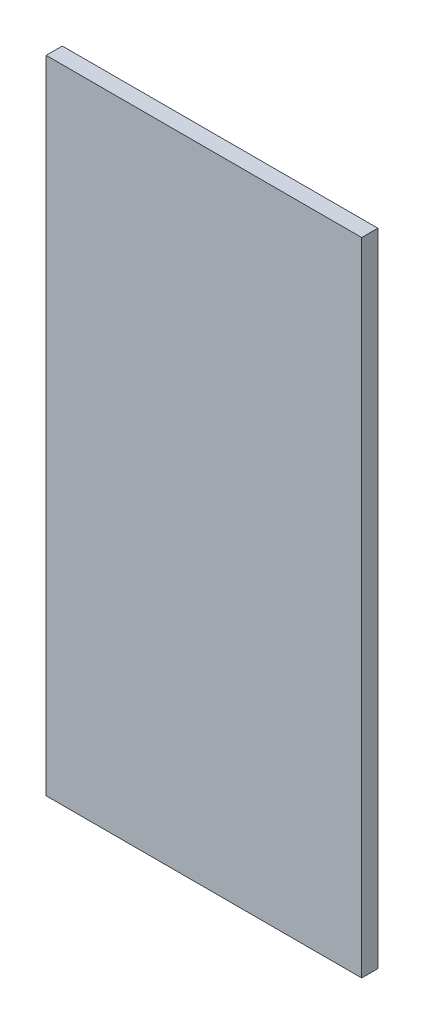
# Autodesk Inventor part: door
Saved by Autodesk Inventor 2023 (Build 270158000, 158)
## iProperties
Created: 2023-04-03
Part Number: door
Material: Generic
Document SubType Name: Modeling
Designer: shrey
Density: 1 g/cm^3
Appearance: Default
Author: shrey
Autodesk Inventor part; units mm, degrees
ref_plane "YZ Plane" through (0, 0, 0) normal (1, 0, 0) x (0, 1, 0)
ref_plane "XZ Plane" through (0, 0, 0) normal (0, 1, 0) x (-1, 0, 0)
ref_plane "XY Plane" through (0, 0, 0) normal (0, 0, 1) x (1, 0, 0)
ref_plane "Work Plane1" through (35.594, 304.8, 19.7663) normal (0, 1, 0) x (-1, 0, 0)
sketch "Sketch1" plane through (35.594, 304.8, 19.7663) normal (0, 1, 0) x (-1, 0, 0)
  line L0 (38.594, -19.7663) -> (338.594, -19.7663)
  line L1 (338.594, -19.7663) -> (338.594, -4.4065)
  line L2 (338.594, -4.4065) -> (38.594, -4.4065)
  line L3 (38.594, -4.4065) -> (38.594, -19.7663)
  line L4 (-28.594, 8.7337) -> (-18.6905, 8.7337) projected
  line L5 (-18.6905, 8.7337) -> (-18.6905, 7.8485) projected
  spline S0 degree 4 poles (-18.6905, 7.8485) (-15.5521, 7.5495) (-7.3401, 9.7663) (-0.7334, 3.3877) (4.6646, 4.702) (6.2676, 4.9792) knots 0 0 0 0 0 0.558486 0.866888 0.866888 0.866888 0.866888 0.866888 projected
  line L6 (6.2676, 4.9792) -> (8.6213, 4.8047) projected
  line L7 (8.6213, 4.8047) -> (8.6213, 3.7665) projected
  line L8 (8.6213, 3.7665) -> (12.5268, 3.3702) projected
  spline S1 degree 2 poles (12.5268, 3.3702) (17.0414, 4.6064) (21.5535, 3.0659) knots 0 0 0 1 1 1 projected
  spline S2 degree 2 poles (21.5535, 3.0659) (24.6084, 3.7058) (28.594, 2.5935) knots 0 0 0 1 1 1 projected
  line L9 (28.594, 2.5935) -> (28.594, -4.4065) projected
  line L10 (28.594, -4.4065) -> (35.594, -4.4065) projected
  line L11 (35.594, -4.4065) -> (35.594, -19.7663) projected
  line L12 (35.594, -19.7663) -> (-139.594, -19.7663) projected
  line L13 (-139.594, -19.7663) -> (-139.594, -9.7663) projected
  line L14 (-139.594, -9.7663) -> (-28.594, -9.7663) projected
  line L15 (-28.594, -9.7663) -> (-28.594, 8.7337) projected
  point P0 (338.594, -12.0864)
  point P1 (38.594, -12.0864)
  dimension "d0" = 3
  dimension "d1" = 300
  constraints: 8 end point, 3 parallel, 2 midpoint, 1 collinear, 1 horizontal, 1 perpendicular
  measures "d0" distance of L0.start L11.end
  measures "d1" distance of point (338.594, -12.086) point (38.594, -12.086)
ref_plane "Work Plane2" through (0, -304.8, 0) normal (0, -1, 0) x (1, 0, 0)
extrude "Extrusion1" add sketch "Sketch1" against normal up to surface (609.6 mm away) contours L3 L2 L1 L0
body "Solid1"
